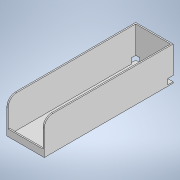
# Autodesk Inventor part: Hopper
Saved by Autodesk Inventor 2022 (Build 260153000, 153)
## iProperties
Created: 2022-01-17
Part Number: Hopper
Material: Generic
Document SubType Name: Modeling
Designer: Work
Density: 1 g/cm^3
Appearance: Default
Author: Work
Autodesk Inventor part; units mm, degrees
ref_plane "YZ Plane" through (0, 0, 0) normal (1, 0, 0) x (0, 1, 0)
ref_plane "XZ Plane" through (0, 0, 0) normal (0, 1, 0) x (-1, 0, 0)
ref_plane "XY Plane" through (0, 0, 0) normal (0, 0, 1) x (1, 0, 0)
sketch "Sketch1" plane through (0, 0, 0) normal (0, 0, 1) x (1, 0, 0)
  line L0 (0, 0) -> (87.28, 0)
  line L1 (0, 0) -> (0, 15.7)
  line L2 (87.28, 0) -> (87.28, 15.7)
  line L3 (87.28, 15.7) -> (0, 15.7)
  dimension "d0" = 87.28
  dimension "d1" = 15.7
  dimension "d2" = 15.7
  constraints: 8 end point, 2 vertical, 1 horizontal
  measures "d0" distance of L0.start L0.end
  measures "d1" distance of L0.start L1.end
  measures "d2" distance of L0.end L2.end
extrude "Extrusion1" add sketch "Sketch1" along normal blind 3
sketch "Sketch2" plane through (0, 0, 0) normal (0, -1, 0) x (1, 0, 0)
  line L0 (87.28, 0) -> (0, 0)
  line L1 (0, 0) -> (0, -297.64)
  line L2 (0, -297.64) -> (87.28, -297.64)
  line L3 (87.28, -297.64) -> (87.28, 0)
  dimension "d5" = 297.64
  constraints: 8 end point, 2 coincident, 2 parallel, 1 horizontal, 1 perpendicular
  measures "d5" distance of L1.end L0.end
extrude "Extrusion2" add sketch "Sketch2" against normal blind 3
sketch "Sketch3" plane through (87.28, 0, 3) normal (1, 0, 0) x (0, 0, -1)
  line L0 (0, 15.7) -> (0, 79.2)
  line L1 (0, 79.2) -> (3, 79.2)
  line L2 (3, 15.7) -> (0, 15.7) projected
  line L3 (3, 79.2) -> (3, 15.7)
  line L4 (3, 3) -> (3, 15.7) projected
  line L5 (3, 15.7) -> (3, 3)
  line L6 (3, 3) -> (300.64, 3)
  line L7 (300.64, 3) -> (300.64, 79.2)
  line L8 (300.64, 79.2) -> (3, 79.2)
  point P0 (3, 0)
  dimension "d8" = 63.5
  constraints: 14 end point, 4 perpendicular, 2 vertical, 1 coincident, 1 horizontal
  measures "d8" distance of L0.start L0.end
extrude "Extrusion3" add sketch "Sketch3" against normal blind 3
fillet "Fillet1" radius 20 1 edges at (85.78, 79.2, 3)
sketch "Sketch4" plane through (0, 0, 3) normal (-1, 0, 0) x (0, 0, 1)
  line L0 (0, 0) -> (0, 59.2) projected
  line L1 (0, 15.7) -> (0, 79.2)
  line L2 (0, 79.2) -> (-3, 79.2)
  line L3 (0, 15.7) -> (-3, 15.7) projected
  line L4 (-3, 79.2) -> (-3, 15.7)
  line L5 (-3, 15.7) -> (-3, 3) projected
  line L6 (-3, 15.7) -> (-3, 3)
  line L7 (-3, 3) -> (-300.64, 3)
  line L8 (-300.64, 0) -> (-300.64, 79.2) projected
  line L9 (-300.64, 79.2) -> (-300.64, 3)
  line L10 (-300.64, 79.2) -> (-3, 79.2)
  point P0 (-3, 0)
  dimension "d12" = 63.5
  dimension "d13" = 3
  constraints: 14 end point, 2 collinear, 2 perpendicular, 2 point on line, 1 horizontal, 1 vertical
  measures "d12" distance of L1.start L1.end
  measures "d13" distance of L1.end L2.end
extrude "Extrusion4" add sketch "Sketch4" against normal blind 3
fillet "Fillet2" radius 20 1 edges at (1.5, 79.2, 3)
sketch "Sketch5" plane through (87.28, 0, -297.64) normal (0, 0, -1) x (-1, 0, 0)
  line L0 (0, 79.2) -> (3, 79.2) projected
  line L1 (3, 3) -> (84.28, 3) projected
  line L2 (3, 79.2) -> (84.28, 79.2)
  line L3 (84.28, 79.2) -> (84.28, 3)
  line L4 (84.28, 3) -> (3, 3)
  line L5 (3, 3) -> (3, 79.2)
  point P0 (87.28, 0)
  constraints: 8 end point, 2 parallel, 1 horizontal, 1 perpendicular
extrude "Extrusion5" add sketch "Sketch5" against normal blind 3
sketch "Sketch6" plane through (87.28, 0, 3) normal (1, 0, 0) x (0, 0, -1)
  line L0 (300.64, 0) -> (300.64, 79.2) projected
  line L1 (300.64, 3) -> (288.125, 3)
  line L2 (300.64, 0) -> (0, 0) projected
  line L3 (300.64, 3) -> (300.64, 15.7)
  line L4 (288.125, 3) -> (288.125, 15.7)
  line L5 (288.125, 15.7) -> (300.64, 15.7)
  point P0 (3, 0)
  dimension "d19" = 3
  dimension "d20" = 12.515
  dimension "d21" = 12.7
  constraints: 8 end point, 2 horizontal, 2 point on line, 1 vertical
  measures "d19" distance between parallel lines of L2 L1
  measures "d20" distance of L1.start L1.end
  measures "d21" distance of L1.start L3.end
extrude "Extrusion6" cut sketch "Sketch6" against normal blind 3
sketch "Sketch7" plane through (87.28, 0, -297.64) normal (0, 0, -1) x (-1, 0, 0)
  line L0 (0, 15.7) -> (3, 15.7) projected
  line L1 (3, 15.7) -> (12.515, 15.7)
  line L2 (3, 15.7) -> (84.28, 15.7) projected
  line L3 (12.515, 15.7) -> (12.515, 3)
  line L4 (3, 3) -> (84.28, 3) projected
  line L5 (0, 3) -> (3, 3) projected
  line L6 (3, 3) -> (12.515, 3)
  line L7 (3, 15.7) -> (3, 3) projected
  line L8 (3, 15.7) -> (3, 3)
  point P0 (87.28, 0)
  dimension "d24" = 9.515
  constraints: 8 end point, 2 point on line, 1 collinear, 1 perpendicular, 1 vertical
  measures "d24" distance of L0.end L1.end
extrude "Extrusion7" cut sketch "Sketch7" against normal blind 3
sketch "Sketch8" plane through (87.28, 0, -297.64) normal (0, 0, -1) x (-1, 0, 0)
  line L0 (87.28, 0) -> (87.28, 79.2) projected
  line L1 (87.28, 3) -> (74.765, 3)
  line L2 (87.28, 0) -> (0, 0) projected
  line L3 (74.765, 3) -> (74.765, 15.7)
  line L4 (74.765, 15.7) -> (87.28, 15.7)
  line L5 (87.28, 15.7) -> (87.28, 3)
  dimension "d27" = 3
  dimension "d28" = 12.515
  dimension "d29" = 12.7
  constraints: 8 end point, 2 point on line, 1 collinear, 1 horizontal, 1 perpendicular, 1 vertical
  measures "d27" distance between parallel lines of L2 L1
  measures "d28" distance of L1.start L1.end
  measures "d29" distance of L1.end L3.end
extrude "Extrusion8" cut sketch "Sketch8" against normal blind 3
sketch "Sketch9" plane through (0, 0, -297.64) normal (-1, 0, 0) x (0, 0, 1)
  line L0 (0, 15.7) -> (3, 15.7) projected
  line L1 (3, 3) -> (3, 15.7) projected
  line L2 (3, 15.7) -> (3, 3)
  line L3 (12.515, 15.7) -> (0, 15.7) projected
  line L4 (3, 15.7) -> (12.515, 15.7)
  line L5 (12.515, 15.7) -> (12.515, 3) projected
  line L6 (12.515, 15.7) -> (12.515, 3)
  line L7 (12.515, 3) -> (3, 3)
  point P0 (297.64, 0)
  constraints: 8 end point, 2 collinear, 1 perpendicular, 1 vertical
extrude "Extrusion9" cut sketch "Sketch9" against normal blind 3
sketch "Sketch10" plane through (0, 3, 0) normal (0, 1, 0) x (1, 0, 0)
  circle A0 centre (10, 7) radius 2.125
  circle A1 centre (77.28, 7) radius 2.125
  circle A2 centre (10, 287.64) radius 2.125
  circle A3 centre (77.28, 287.64) radius 2.125
  line L0 (0, 297.64) -> (12.515, 297.64) projected
  line L1 (0, 285.125) -> (0, 297.64) projected
  line L2 (87.28, 297.64) -> (87.28, 285.125) projected
  line L3 (74.765, 297.64) -> (87.28, 297.64) projected
  line L4 (0, -3) -> (87.28, -3) projected
  line L5 (0, 297.64) -> (0, -3) projected
  line L6 (87.28, 297.64) -> (87.28, -3) projected
  point P0 (0, 0)
  dimension "d34" = 4.25
  dimension "d35" = 4.25
  dimension "d36" = 4.25
  dimension "d37" = 4.25
  dimension "d38" = 10
  dimension "d39" = 10
  dimension "d40" = 10
  dimension "d41" = 10
  dimension "d42" = 10
  dimension "d43" = 10
  dimension "d44" = 10
  dimension "d45" = 10
  constraints: 4 centre point
  measures "d34" diameter of A0
  measures "d35" diameter of A1
  measures "d36" diameter of A2
  measures "d37" diameter of A3
  measures "d38" distance from line of A2.centre L0
  measures "d39" distance from line of L1 A2.centre
  measures "d40" distance from line of L2 A3.centre
  measures "d41" distance from line of A3.centre L3
  measures "d42" distance from line of L4 A0.centre
  measures "d43" distance from line of L5 A0.centre
  measures "d44" distance from line of L4 A1.centre
  measures "d45" distance from line of L6 A1.centre
extrude "Extrusion10" cut sketch "Sketch10" against normal blind 3
body "Solid1"
